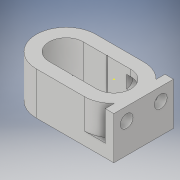
# Autodesk Inventor part: bedtiedown3
Saved by Autodesk Inventor 2019.1 (Build 231200000, 200)
## iProperties
Created: 2019-08-29
Part Number: bedtiedown3
Material: Generic
Document SubType Name: Modeling
Designer: Computus
Density: 1 g/cm^3
Appearance: Default
Author: Computus
## iProperties of the stored document bedtiedown2_3DPrint.ipt
Created: 2019-08-30
Part Number: bedtiedown2_3DPrint
Material: Generic
Document SubType Name: Modeling
Designer: Computus
Density: 1 g/cm^3
Appearance: Default
Author: Computus
Autodesk Inventor part; units mm, degrees
ref_plane "YZ Plane" through (0, 0, 0) normal (1, 0, 0) x (0, 1, 0)
ref_plane "XZ Plane" through (0, 0, 0) normal (0, 1, 0) x (-1, 0, 0)
ref_plane "XY Plane" through (0, 0, 0) normal (0, 0, 1) x (1, 0, 0)
sketch "Sketch1" plane through (0, 0, 0) normal (0, 1, 0) x (-1, 0, 0)
  arc A0 (0, 4) -> (0, -4) centre (0, 0) ccw
  arc A1 (11.1938, -4) -> (11.1938, 4) centre (11.1938, 0) ccw
  line L0 (11.1938, -4) -> (0, -4)
  line L1 (11.1938, 4) -> (0, 4)
  line L2 (11.1938, -7) -> (0, -7)
  line L3 (0, 7) -> (11.1938, 7)
  arc A2 (5.5969, 4.2041) -> (5.4492, 4) centre (11.1938, 0) ccw
  arc A3 (5.7446, 4) -> (5.5969, 4.2041) centre (0, 0) ccw
  arc A4 (5.4492, -4) -> (5.5969, -4.2041) centre (11.1938, 0) ccw
  arc A5 (11.1938, -7) -> (11.1938, 7) centre (11.1938, 0) ccw
  arc A6 (0, 7) -> (0, -7) centre (0, 0) ccw
  arc A7 (5.5969, -4.2041) -> (5.7446, -4) centre (0, 0) ccw
  dimension "d0" = 8
  dimension "d1" = 8
  constraints: 16 point on circle, 8 centre point, 8 end point, 6 tangent, 4 point on line, 3 coincident, 1 parallel
  measures "d0" diameter of A0
  measures "d1" diameter of A1
extrude "Extrusion1" add sketch "Sketch1" along normal blind 10
sketch "Sketch2" plane through (0, 0, 0) normal (0, -1, 0) x (1, 0, 0)
  arc A0 (0, -7) -> (0, 7) centre (0, 0) ccw
  arc A1 (0, -4) -> (0, 4) centre (0, 0) ccw
  line L0 (0, -7) -> (0, -4)
  line L1 (0, 4) -> (0, 7)
  line L2 (0, -7) -> (-11.1938, -7) projected
  line L3 (0, -7) -> (5, -7)
  arc A2 (0, -7) -> (0, 7) centre (0, 0) ccw projected
  line L4 (0, 7) -> (5, 7)
  line L5 (5, 7) -> (5, -7)
  dimension "d6" = 5
  constraints: 10 end point, 4 point on circle, 3 tangent, 2 centre point, 2 coincident, 2 horizontal, 2 vertical, 1 perpendicular
  measures "d6" distance of L0.start L3.end
extrude "Extrusion2" add sketch "Sketch2" against normal blind 3 contours L0 A1 L1 A0 L5 | A0 L5 L3 | A0 L4 L5
sketch "Sketch3" plane through (5, 0, 7) normal (1, 0, 0) x (0, 0, -1)
  line L0 (14, 10) -> (0, 10) projected
  line L1 (0, 0) -> (14, 0)
  line L2 (14, 0) -> (14, 10)
  line L3 (14, 10) -> (0, 10)
  line L4 (0, 10) -> (0, 0)
  point P0 (7, 0)
  constraints: 8 end point, 2 parallel, 1 horizontal, 1 perpendicular
extrude "Extrusion3" add sketch "Sketch3" along normal blind 2
sketch "Sketch4" plane through (7, 0, 7) normal (1, 0, 0) x (0, 0, -1)
  circle A0 centre (3, 7) radius 1.5
  circle A1 centre (11, 7) radius 1.5
  line L0 (14, 10) -> (0, 10) projected
  line L1 (0, 10) -> (0, 0) projected
  line L2 (14, 0) -> (14, 10) projected
  point P0 (7, 0)
  dimension "d11" = 3
  dimension "d12" = 3
  dimension "d13" = 3
  dimension "d14" = 3
  dimension "d15" = 3
  dimension "d16" = 3
  constraints: 2 centre point
  measures "d11" diameter of A0
  measures "d12" diameter of A1
  measures "d13" distance from line of L0 A1.centre
  measures "d14" distance from line of L0 A0.centre
  measures "d15" distance from line of A0.centre L1
  measures "d16" distance from line of A1.centre L2
extrude "Extrusion4" cut sketch "Sketch4" against normal blind 8
sketch "Sketch5" plane through (0, 10, 0) normal (0, 1, 0) x (1, 0, 0)
  point P0 (0, 0)
sketch "Sketch6" plane through (0, 10, 0) normal (0, 1, 0) x (1, 0, 0)
  point P0 (0, 0)
body "Solid1"
